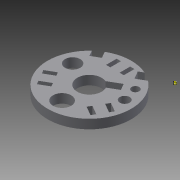
# Autodesk Inventor part: Gripper V 10.0 base 6mm
Saved by Autodesk Inventor 2015 (Build 190159000, 159)
## iProperties
Created: 2015-06-11
Part Number: Gripper V 10.0 base 6mm
Material: Generic
Document SubType Name: Modeling
Designer: Stackpole
Density: 1 g/cm^3
Appearance: Default
Author: Stackpole
Autodesk Inventor part; units mm, degrees
ref_plane "YZ Plane" through (0, 0, 0) normal (1, 0, 0) x (0, 1, 0)
ref_plane "XZ Plane" through (0, 0, 0) normal (0, 1, 0) x (-1, 0, 0)
ref_plane "XY Plane" through (0, 0, 0) normal (0, 0, 1) x (1, 0, 0)
sketch "Sketch2" plane through (0, 0, 0) normal (0, 0, 1) x (1, 0, 0)
  circle A0 centre (0, 0) radius 27.5
  circle A1 centre (0, 0) radius 8
  dimension "d0" = 55
  dimension "d1" = 16
  constraints: 2 centre point, 1 coincident, 1 concentric
  measures "d0" diameter of A0
  measures "d1" diameter of A1
extrude "Extrusion1" add sketch "Sketch2" along normal blind 6
sketch "Sketch3" plane through (0, 0, 6) normal (0, 0, 1) x (1, 0, 0)
  circle A0 centre (0, 0) radius 22.5 construction
  circle A1 centre (0, 0) radius 27.5 projected
  line L0 (-5.87, 23.8) -> (-3.07, 23.8)
  line L1 (-3.07, 23.8) -> (-3.07, 16.8)
  line L2 (-3.07, 16.8) -> (-5.87, 16.8)
  line L3 (-5.87, 16.8) -> (-5.87, 23.8)
  line L4 (0, 0) -> (0, 27.8091) construction
  line L5 (3.07, 23.8) -> (5.87, 23.8)
  line L6 (5.87, 23.8) -> (5.87, 16.8)
  line L7 (5.87, 16.8) -> (3.07, 16.8)
  line L8 (3.07, 16.8) -> (3.07, 23.8)
  line L9 (-17.6764, -16.9836) -> (-19.0764, -14.5587)
  line L10 (-19.0764, -14.5587) -> (-13.0142, -11.0587)
  line L11 (-13.0142, -11.0587) -> (-11.6142, -13.4836)
  line L12 (-11.6142, -13.4836) -> (-17.6764, -16.9836)
  line L13 (-22.1464, -9.2413) -> (-23.5464, -6.8164)
  line L14 (-23.5464, -6.8164) -> (-17.4842, -3.3164)
  line L15 (-17.4842, -3.3164) -> (-16.0842, -5.7413)
  line L16 (-16.0842, -5.7413) -> (-22.1464, -9.2413)
  line L17 (23.5464, -6.8164) -> (22.1464, -9.2413)
  line L18 (22.1464, -9.2413) -> (16.0842, -5.7413)
  line L19 (16.0842, -5.7413) -> (17.4842, -3.3164)
  line L20 (17.4842, -3.3164) -> (23.5464, -6.8164)
  line L21 (19.0764, -14.5587) -> (17.6764, -16.9836)
  line L22 (17.6764, -16.9836) -> (11.6142, -13.4836)
  line L23 (11.6142, -13.4836) -> (13.0142, -11.0587)
  line L24 (13.0142, -11.0587) -> (19.0764, -14.5587)
  line L25 (0, 27.5) -> (22.8099, 27.5) construction
  circle A2 centre (0, 0) radius 27.5 projected
  dimension "d4" = 5
  dimension "d5" = 2.8
  dimension "d6" = 7
  dimension "d9" = 2.8
  dimension "d10" = 7
  dimension "d12" = 3.07
  dimension "d13" = 3.07
  dimension "d16" = 360
  dimension "d20" = 3.7
  constraints: 52 end point, 4 parallel, 3 horizontal, 2 perpendicular, 1 centre point, 1 coincident, 1 collinear, 1 point on line, 1 tangent, 1 vertical, 1 vertical alignment, 50 other
  measures "d5" distance of L1.end L2.end
  measures "d6" distance of L2.end L0.start
  measures "d9" distance of L6.end L7.end
  measures "d10" distance of L5.end L6.end
  measures "d12" distance between parallel lines of L4 L8
  measures "d13" distance between parallel lines of L1 L4
  measures "d20" distance between parallel lines of L25 L0
extrude "Extrusion2" cut sketch "Sketch3" against normal blind 6 contours L0 L1 L2 L3 | L5 L6 L7 L8 | L9 L10 L11 L12 | L13 L14 L15 L16 | L17 L18 L19 L20 | L21 L22 L23 L24
sketch "Sketch7" plane through (0, 0, 6) normal (0, 0, 1) x (1, 0, 0)
  line L0 (19.5793, 23.0548) -> (11.3521, 18.3048)
  line L1 (11.3521, 18.3048) -> (8.3521, 23.501)
  line L2 (8.3521, 23.501) -> (16.5793, 28.251)
  line L3 (16.5793, 28.251) -> (19.5793, 23.0548)
  line L4 (23.5464, -6.8164) -> (5.87, 23.8) construction
  line L5 (5.87, 23.8) -> (16.4282, 29.8958) construction
  arc A0 (27.5, 0) -> (27.5, 0) centre (0, 0) ccw projected
  dimension "d16" = 360
  dimension "d59" = 6
  dimension "d60" = 9.5
  dimension "d100" = 2
  dimension "d101" = 1.5
  constraints: 12 end point, 4 perpendicular, 1 coincident, 1 parallel
  measures "d59" distance of L2.end L0.start
  measures "d60" distance of L1.end L2.end
  measures "d100" distance between parallel lines of L4 L1
  measures "d101" distance between parallel lines of L5 L2
extrude "Extrusion6" cut sketch "Sketch7" against normal blind 10 contours L0 A0 L2 L3 | L0 L1 L2 A0 picked at (10.9756, 21.9728)
sketch "Sketch6" plane through (0, 0, 6) normal (0, 0, 1) x (1, 0, 0)
  line L0 (23.5464, -6.8164) -> (5.87, 23.8) construction
  line L1 (-16.4532, 16.4649) -> (-19.4532, 21.6611)
  line L2 (-19.4532, 21.6611) -> (-14.2571, 24.6611)
  line L3 (-14.2571, 24.6611) -> (-11.2571, 19.4649)
  line L4 (-11.2571, 19.4649) -> (-16.4532, 16.4649)
  line L5 (-5.87, 16.8) -> (-5.87, 23.8) projected
  line L6 (-5.87, 23.8) -> (-7.957, 25.0049) construction
  line L7 (-23.5464, -6.8164) -> (-5.87, 23.8) construction
  circle A0 centre (0, 0) radius 27.5 projected
  line L8 (10.8086, 11.7395) -> (13.3086, 7.4094)
  circle A1 centre (0, 0) radius 8 projected
  line L9 (5.87, 23.8) -> (-0.452, 20.15) construction
  line L10 (13.3086, 7.4094) -> (0.9952, 0.3002)
  line L11 (10.8086, 11.7395) -> (-2.1818, 4.2395)
  line L12 (-2.1818, 4.2395) -> (0.9952, 0.3002)
  line L13 (17.0369, 21.5869) -> (11.3521, 18.3048) projected
  line L14 (11.3521, 18.3048) -> (8.3521, 23.501) projected
  dimension "d47" = 6
  dimension "d48" = 6
  dimension "d71" = 5
  dimension "d84" = 15.2302
  dimension "d96" = 14.2183
  dimension "d97" = 15
  dimension "d102" = 5.414
  dimension "d103" = 12.3093
  dimension "d104" = 19
  constraints: 24 end point, 5 perpendicular, 1 other
  measures "d47" distance of L1.end L2.end
  measures "d48" distance of L2.end L3.end
  measures "d71" distance of L8.start L8.end
  measures "d84" distance from line of point (0, 0) L8
  measures "d96" distance of L8.end L10.end
  measures "d97" distance of L8.start L11.end
  measures "d102" distance between parallel lines of L13 L11
  measures "d103" distance between parallel lines of L4 L13
  measures "d104" distance between parallel lines of L14 L3
extrude "Extrusion7" cut sketch "Sketch6" against normal blind 10 contours L1 A0 L3 L4 | L1 L2 L3 A0 | L8 L10 A1 L11 | A1 L10 L12 L11 picked at (-14.9352, 19.1568) picked at (0.6663, 3.9594)
fillet "Fillet4" radius 0.3 2 edges at (3.1856, 7.3384, 3) (7.0439, 3.7925, 3)
sketch "Sketch13" plane through (0, 0, 6) normal (0, 0, 1) x (1, 0, 0)
  circle A0 centre (0, -18.0231) radius 6
  circle A1 centre (-17.6976, 6.6203) radius 5
  circle A2 centre (20.25, 3) radius 3.25
  circle A3 centre (17.6614, 12.6185) radius 2.5
  line L0 (-11.6142, -13.4836) -> (-17.6764, -16.9836) projected
  line L1 (17.6764, -16.9836) -> (11.6142, -13.4836) projected
  line L2 (-23.5464, -6.8164) -> (-17.4842, -3.3164) projected
  line L3 (-5.87, 16.8) -> (-5.87, 23.8) projected
  line L4 (-16.4532, 16.4649) -> (-18.6273, 20.2305) projected
  point P0 (0, 0)
  dimension "d146" = 12
  dimension "d147" = 6.5
  dimension "d148" = 10
  dimension "d151" = 5
  dimension "d154" = 9.7385
  dimension "d155" = 9.7385
  dimension "d156" = 8.7122
  dimension "d158" = 6
  constraints: 4 centre point
  measures "d146" diameter of A0
  measures "d147" diameter of A2
  measures "d148" diameter of A1
  measures "d151" diameter of A3
  measures "d154" distance from line of L0 A0.centre
  measures "d155" distance from line of L1 A0.centre
  measures "d156" distance from line of A1.centre L2
  measures "d158" distance from line of A1.centre L4
extrude "Extrusion16" cut sketch "Sketch13" against normal blind 10
body "Solid1"
